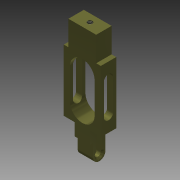
# Autodesk Inventor part: 13_1087_004
Saved by Autodesk Inventor 2014 (Build 180170000, 170)
## iProperties
Created: 2013-08-01
Part Number: 13_1087_004
Material: Titan
Document SubType Name: Modeling
Designer: vogel
Density: 4.51 g/cm^3
Appearance: Titan
Author: vogel
Autodesk Inventor part; units mm, degrees
ref_plane "YZ Plane" through (0, 0, 0) normal (1, 0, 0) x (0, 1, 0)
ref_plane "XZ Plane" through (0, 0, 0) normal (0, 1, 0) x (-1, 0, 0)
ref_plane "XY Plane" through (0, 0, 0) normal (0, 0, 1) x (1, 0, 0)
sketch "Skizze1" plane through (0, 0, 0) normal (0, 0, 1) x (1, 0, 0)
  line L0 (-8.4, 0) -> (8.4, 0) projected
  line L1 (0, -3.5) -> (0, 3.5) projected
  line L2 (-6, 2.5) -> (6, 2.5)
  line L3 (6, 2.5) -> (6, -2.5)
  line L4 (6, -2.5) -> (-6, -2.5)
  line L5 (-6, -2.5) -> (-6, 2.5)
  point P0 (0, 0)
  dimension "d0" = 12
  dimension "d1" = 5
  constraints: 8 end point, 2 parallel, 1 horizontal, 1 perpendicular, 2 other
  measures "d0" distance of L3.end L4.end
  measures "d1" distance of L4.end L2.start
extrude "Extrusion1" add sketch "Skizze1" along normal blind 28
sketch "Skizze2" plane through (-6, 2.5, 0) normal (0, 1, 0) x (1, 0, 0)
  line L0 (0, -28) -> (1.5, -28)
  line L1 (1.5, -28) -> (1.5, -20)
  line L2 (1.5, -20) -> (0, -20)
  line L3 (0, -20) -> (0, -28)
  line L4 (12, -28) -> (10.5, -28)
  line L5 (10.5, -28) -> (10.5, -20)
  line L6 (10.5, -20) -> (12, -20)
  line L7 (12, -20) -> (12, -28)
  line L8 (-2.4, 0) -> (14.4, 0) projected
  line L9 (6, 5.6) -> (6, -33.6) projected
  point P0 (6, 0)
  dimension "d4" = 9
  dimension "d5" = 8
  constraints: 16 end point, 4 parallel, 2 horizontal, 2 perpendicular, 1 collinear, 1 other
  measures "d4" distance between parallel lines of L5 L1
  measures "d5" distance of L4.end L5.end
extrude "Extrusion2" cut sketch "Skizze2" against normal through all
sketch "Skizze3" plane through (0, 0, 0) normal (0, 0, -1) x (-1, 0, 0)
  line L0 (6, 2.5) -> (-6, 2.5) projected
  line L1 (-2.5, 2.5) -> (2.5, 2.5)
  line L2 (2.5, 2.5) -> (2.5, -1.5)
  line L3 (2.5, -1.5) -> (-2.5, -1.5)
  line L4 (-2.5, -1.5) -> (-2.5, 2.5)
  line L5 (8.4, 0) -> (-8.4, 0) projected
  line L6 (0, -3.5) -> (0, 3.5) projected
  point P0 (0, 0)
  dimension "d8" = 5
  dimension "d9" = 4
  constraints: 8 end point, 2 parallel, 1 horizontal, 1 perpendicular, 1 point on line, 1 other
  measures "d8" distance of L2.end L3.end
  measures "d9" distance between parallel lines of L0 L3
extrude "Extrusion3" add sketch "Skizze3" along normal blind 10
sketch "Skizze5" plane through (0, 0, 28) normal (0, 0, 1) x (1, 0, 0)
  line L0 (-4.5, 2.5) -> (-4.5, -2.5) projected
  line L1 (-4.5, -2.5) -> (4.5, -2.5) projected
  line L2 (4.5, -2.5) -> (4.5, 2.5) projected
  line L3 (4.5, 2.5) -> (-4.5, 2.5) projected
  line L4 (-4.5, 0) -> (4.5, 0)
  line L5 (0, 2.5) -> (0, -2.5)
  point P0 (0, 0)
  point P1 (0, 0)
  constraints: 4 end point, 4 midpoint, 1 coincident
hole "Bohrung2" at (0, 0, 28) direction (0, 0, -1) diameter 1.567 depth 6 tip angle 118 thread size "M2x0.4" class "6H" standard "ISO Metric profile"
sketch "Skizze6" plane through (2.5, -1.5, 0) normal (1, 0, 0) x (0, 0, -1)
  line L0 (0, 0) -> (0, 4) projected
  line L1 (10, 4) -> (10, 0) projected
  line L2 (10, 2) -> (0, 2)
  point P0 (0, 1.5)
  point P1 (8, 2)
  dimension "d28" = 2
  constraints: 2 end point, 2 midpoint, 1 point on line
  measures "d28" distance from line of L1 point (8, 2)
hole "Bohrung3" at (2.5, 0.5, -8) direction (-1, 0, 0) diameter 2 end through all countersink diameter 3 countersink angle 90
sketch "Skizze7" plane through (2.5, -1.5, 0) normal (1, 0, 0) x (0, 0, -1)
  circle A0 centre (8, 2) radius 1.5 projected
  line L0 (0, 0) -> (0, 4) projected
  line L1 (0, 0) -> (10, 0) projected
  line L2 (10, 4) -> (10, 0) projected
  line L3 (2, 2) -> (8, 2) construction
  line L4 (2, 3) -> (8, 3)
  line L5 (8, 1) -> (2, 1)
  arc A1 (2, 3) -> (2, 1) centre (2, 2) ccw
  arc A2 (8, 1) -> (8, 3) centre (8, 2) ccw
  point P0 (0, 1.5)
  point P1 (5, 2)
  dimension "d36" = 2
  dimension "d37" = 2
  dimension "d38" = 2
  constraints: 8 end point, 4 point on circle, 4 tangent, 2 centre point, 2 parallel, 1 midpoint
  measures "d36" distance from line of L3.end L2
  measures "d37" distance from line of L3.start L0
  measures "d38" distance between parallel lines of L4 L5
extrude "Extrusion4" cut sketch "Skizze7" against normal through all contours L4 A2 L5 A0 | A0 L5 A1 L4 picked at (7.5, 2)
sketch "Skizze8" plane through (-2.5, -1.5, 0) normal (0, -1, 0) x (1, 0, 0)
  line L0 (5, 0) -> (5, -10) projected
  line L1 (0, 0) -> (5, 0)
  line L2 (5, 0) -> (5, -4)
  line L3 (5, -4) -> (0, -4)
  line L4 (0, -4) -> (0, 0)
  point P0 (2.5, 0)
  dimension "d41" = 4
  constraints: 8 end point, 2 parallel, 1 horizontal, 1 perpendicular, 1 point on line
  measures "d41" distance between parallel lines of L1 L3
extrude "Extrusion5" add sketch "Skizze8" along normal blind 1
sketch "Skizze9" plane through (-2.5, -2.5, 0) normal (-1, 0, 0) x (0, 0, 1)
  arc A0 (-8, 4) -> (-8, 2) centre (-8, 3) ccw projected
  point P0 (0, 2.5)
hole "Bohrung4" at (-2.5, 0.5, -8) direction (1, 0, 0) diameter 2 end through all countersink diameter 3 countersink angle 90
fillet "Rundung1" radius 2 2 edges at (0, -1.5, -10) (0, 2.5, -10)
sketch "Skizze11" plane through (6, -2.5, 0) normal (1, 0, 0) x (0, 0, -1)
  line L0 (-20, 5) -> (-20, 0) projected
  line L1 (0, 0) -> (-20, 0) projected
  line L2 (0, 5) -> (0, 0) projected
  line L3 (-15, 2.5) -> (-5, 2.5) construction
  line L4 (-15, 4) -> (-5, 4)
  line L5 (-5, 1) -> (-15, 1)
  arc A0 (-15, 4) -> (-15, 1) centre (-15, 2.5) ccw
  arc A1 (-5, 1) -> (-5, 4) centre (-5, 2.5) ccw
  point P0 (0, 2.5)
  point P1 (-10, 2.5)
  dimension "d61" = 3
  dimension "d62" = 2.5
  dimension "d63" = 5
  dimension "d64" = 5
  constraints: 8 end point, 4 point on circle, 4 tangent, 2 centre point, 2 parallel, 1 midpoint
  measures "d61" distance between parallel lines of L4 L5
  measures "d62" distance between parallel lines of L3 L1
  measures "d63" distance from line of L3.end L2
  measures "d64" distance from line of L3.start L0
extrude "Extrusion6" cut sketch "Skizze11" against normal through all
sketch "Skizze12" plane through (-4.5, -2.5, 28) normal (0, -1, 0) x (1, 0, 0)
  line L0 (-1.5, -28) -> (-1.5, -8) projected
  line L1 (2, -28) -> (-1.5, -28) projected
  line L2 (10.5, -28) -> (10.5, -8) projected
  line L3 (10.5, -8) -> (9, -8) projected
  line L4 (4.5, -13) -> (4.5, -23) construction
  line L5 (0.5, -13) -> (0.5, -23)
  line L6 (8.5, -23) -> (8.5, -13)
  arc A0 (8.5, -13) -> (0.5, -13) centre (4.5, -13) ccw
  arc A1 (0.5, -23) -> (8.5, -23) centre (4.5, -23) ccw
  point P0 (4.5, -28)
  point P1 (4.5, -18)
  dimension "d67" = 6
  dimension "d68" = 8
  dimension "d69" = 5
  dimension "d70" = 5
  constraints: 8 end point, 4 point on circle, 4 tangent, 2 centre point, 2 parallel, 1 midpoint
  measures "d67" distance between parallel lines of L4 L2
  measures "d68" distance between parallel lines of L5 L6
  measures "d69" distance from line of L3 L4.start
  measures "d70" distance from line of L4.end L1
extrude "Extrusion7" cut sketch "Skizze12" against normal through all
